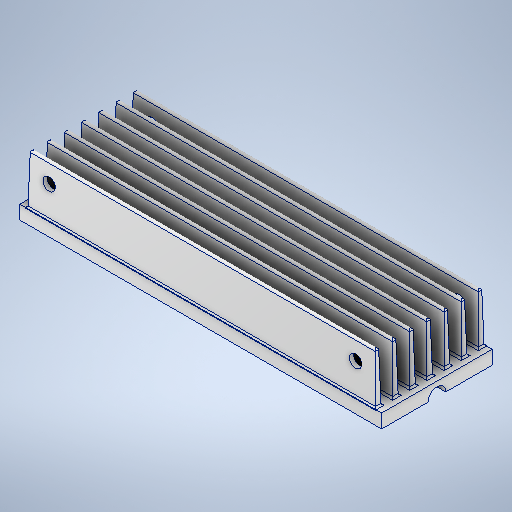
# Autodesk Inventor part: Heat Sink Holed drilled
Saved by Autodesk Inventor 2026.2 (Build 302298010, 298A)
## iProperties
Created: 2026-04-26
Part Number: Heat Sink Holed drilled
Material: Aluminum 6061
Document SubType Name: Modeling
Designer: piete
Density: 2.7 g/cm^3
Appearance: Aluminum - Flat
Author: piete
Autodesk Inventor part; units mm, degrees
ref_plane "YZ Plane" through (0, 0, 0) normal (1, 0, 0) x (0, 1, 0)
ref_plane "XZ Plane" through (0, 0, 0) normal (0, 1, 0) x (-1, 0, 0)
sketch "Sketch1" plane through (0, 0, 0) normal (0, 1, 0) x (-1, 0, 0)
  line L0 (32.75, 10) -> (-32.75, 10)
  line L1 (-32.75, 10) -> (-32.75, -10)
  line L2 (-32.75, -10) -> (32.75, -10)
  line L3 (32.75, -10) -> (32.75, 10)
  point P0 (0, 0)
  dimension "d0" = 65.5
  dimension "d1" = 32.75
  dimension "d2" = 20
  dimension "d3" = 10
  constraints: 8 end point, 2 parallel, 1 horizontal, 1 perpendicular
  measures "d0" distance of L1.end L2.end
  measures "d1" distance from line of point (0, 0) L3
  measures "d2" distance of L2.end L0.start
  measures "d3" distance from line of point (0, 0) L2
extrude "Extrusion1" add sketch "Sketch1" along normal blind 2.5
sketch "Sketch2" plane through (0, 0, 0) normal (1, 0, 0) x (0, 1, 0)
  line L0 (11.2, 0.5) -> (2.5, 0.5)
  line L1 (2.5, 0.5) -> (2.5, -0.5)
  line L2 (2.5, -0.5) -> (11.2, -0.5)
  line L3 (11.2, -0.5) -> (11.2, 0.5)
  line L4 (0, -10) -> (0, 10) projected
  circle A0 centre (11.2, 0) radius 0.3
  circle A1 centre (2.8, -0.8) radius 0.3
  circle A2 centre (2.8, 0.8) radius 0.3
  line L5 (2.5, -10) -> (2.5, 10) projected
  line L6 (2.5, 0.8) -> (2.5, -0.8)
  line L7 (11.2071, -0.2999) -> (2.8, -0.5)
  line L8 (11.2, 0.3) -> (2.8, 0.5)
  point P0 (0, 0)
  point P1 (0, 0)
  point P2 (11.2, 0)
  point P3 (11.2, -0.3001)
  point P4 (11.2, -0.3)
  dimension "d6" = 8.7
  dimension "d7" = 1
  dimension "d8" = 11.2
  dimension "d9" = 0.5
  dimension "d10" = 0.6
  dimension "d11" = 0
  dimension "d12" = 0
  dimension "d13" = 0.6
  dimension "d14" = 0.6
  dimension "d15" = 0.3
  dimension "d16" = 0.3
  dimension "d17" = 0.3
  dimension "d18" = 0.3
  constraints: 14 end point, 6 point on circle, 5 point on line, 3 centre point, 2 midpoint, 2 parallel, 1 horizontal, 1 perpendicular, 1 tangent
  measures "d6" distance of L2.end L1.end
  measures "d7" distance of L1.end L0.end
  measures "d8" distance between parallel lines of L4 L3
  measures "d9" distance from line of point (0, 0) L2
  measures "d10" diameter of A0
  measures "d11" distance of point (11.2, 0) A0.centre
  measures "d12" distance of A0.centre point (11.2, 0)
  measures "d13" diameter of A1
  measures "d14" diameter of A2
  measures "d15" distance from line of L0 A2.centre
  measures "d16" distance from line of L5 A2.centre
  measures "d17" distance from line of L5 A1.centre
  measures "d18" distance from line of L2 A1.centre
extrude "Extrusion2" add sketch "Sketch2" along normal mid plane 63.5 contours L8 A0 L7 L2 L1 L0 | L0 L5 A2 | A0 L3 | L3 A0 | L2 A1 L5
sketch "Sketch3" plane through (0, 0, 0) normal (0, 0, 1) x (1, 0, 0)
  circle A0 centre (30.95, 11.2) radius 0.3
  circle A1 centre (31.75, 2.8) radius 0.3
  line L0 (31.75, 11.2) -> (31.75, 2.8) projected
  line L1 (-32.75, 2.5) -> (32.75, 2.5) projected
  line L2 (31.75, 11.2) -> (31.75, 11.5) projected
  line L3 (-31.75, 11.2) -> (31.75, 11.2) projected
  line L4 (31.25, 11.2) -> (31.4501, 2.7929)
  line L5 (30.95, 11.5) -> (31.75, 11.5)
  line L6 (31.75, 11.5) -> (31.75, 3.1)
  point P0 (0, 0)
  dimension "d21" = 0.6
  dimension "d22" = 0.6
  dimension "d23" = 0
  dimension "d24" = 0.3
  dimension "d25" = 0.8
  dimension "d26" = 8.7
  constraints: 6 end point, 4 point on circle, 2 centre point, 2 point on line, 2 tangent
  measures "d21" diameter of A0
  measures "d22" diameter of A1
  measures "d23" distance from line of L0 A1.centre
  measures "d24" distance from line of L1 A1.centre
  measures "d25" distance from line of L2 A0.centre
  measures "d26" distance from line of L1 A0.centre
extrude "Extrusion3" cut sketch "Sketch3" along normal mid plane 63.5 contours A0 L5 L2 L3 | L3 L0 A1 L4 | A1
mirror "Mirror1" about plane through (0, 0, 0) normal (1, 0, 0) of "Extrusion3"
pattern_linear "Rectangular Pattern1" count 7 spacing 3.11 along (0, 0, 1) of "Extrusion2", "Extrusion3" first direction both ways yes
sketch "Sketch4" plane through (32.75, 0, 10) normal (1, 0, 0) x (0, 0, -1)
  circle A0 centre (10, 0) radius 1.6
  dimension "d32" = 3.2
  constraints: 1 centre point, 1 coincident
  measures "d32" diameter of A0
extrude "Extrusion4" cut sketch "Sketch4" against normal blind 40
pattern_linear "Rectangular Pattern2" count 7 spacing 3.11 along (0, 0, 1) of "Extrusion3", "Mirror1" first direction both ways yes
ref_plane "Work Plane1" through (0, 0, 9.33) normal (0, 0, 1) x (1, 0, 0)
sketch "Sketch5" plane through (0, 0, 9.33) normal (0, 0, 1) x (1, 0, 0)
  circle A0 centre (-27.75, 8) radius 1.1
  line L0 (32.75, 0) -> (-32.75, 0) projected
  line L1 (-32.75, 0) -> (-32.75, 2.5) projected
  circle A1 centre (27.75, 8) radius 1.1
  line L2 (32.75, 0) -> (32.75, 2.5) projected
  point P0 (0, 0)
  dimension "d39" = 2.2
  dimension "d40" = 8
  dimension "d41" = 5
  dimension "d42" = 2.2
  dimension "d43" = 5
  dimension "d44" = 8
  constraints: 2 centre point
  measures "d39" diameter of A0
  measures "d40" distance from line of L0 A0.centre
  measures "d41" distance from line of A0.centre L1
  measures "d42" diameter of A1
  measures "d43" distance from line of L2 A1.centre
  measures "d44" distance from line of L0 A1.centre
extrude "Extrusion5" cut sketch "Sketch5" along normal mid plane 1
mirror "Mirror2" about plane through (0, 0, 0) normal (0, 0, 1) of "Extrusion5"
fillet "Fillet1" radius 1.6 1 edges at (-7.25, 1.6, 0)
equation "\"d1\" = 0.5 * d0"
equation "\"d3\" = 0.5 * d2"
body "Solid1"
